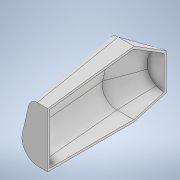
# Autodesk Inventor part: Housing
Saved by Autodesk Inventor 2021 (Build 250183000, 183)
## iProperties
Created: 2022-01-12
Part Number: Housing
Material: Generic
Document SubType Name: Modeling
Designer: stefi
Density: 1 g/cm^3
Appearance: Default
Author: stefi
Autodesk Inventor part; units mm, degrees
ref_plane "YZ Plane" through (0, 0, 0) normal (1, 0, 0) x (0, 1, 0)
ref_plane "XZ Plane" through (0, 0, 0) normal (0, 1, 0) x (-1, 0, 0)
ref_plane "Work Plane1" through (0, 0, 711.2) normal (0, 0, 1) x (1, 0, 0)
sketch "Sketch1" plane through (0, 0, 711.2) normal (0, 0, 1) x (1, 0, 0)
  line L0 (0.7413, 24.2751) -> (0.7413, -22.8249)
  line L1 (0.7413, -22.8249) -> (-11.3287, -22.8249)
  arc A0 (-23.0997, -8.085) -> (-11.3287, -22.8249) centre (-11.3287, -10.7549) ccw
  line L2 (-23.0997, -8.085) -> (-16.8814, 19.3297)
  arc A1 (-10.6887, 24.2751) -> (-16.8814, 19.3297) centre (-10.6887, 17.9251) ccw
  line L3 (-10.6887, 24.2751) -> (0.7413, 24.2751)
  point P0 (0, 0)
  dimension "d1" = 47.1
  dimension "d2" = 12.07
  dimension "d3" = 12.07
  dimension "d4" = 6.35
  dimension "d5" = 11.43
  constraints: 8 end point, 4 point on circle, 4 tangent, 2 centre point, 1 horizontal, 1 perpendicular, 1 vertical
  measures "d1" distance of L0.start L0.end
  measures "d2" distance of L0.end L1.end
  measures "d3" radius of A0
  measures "d4" radius of A1
  measures "d5" distance of L3.start L0.start
ref_plane "Work Plane2" through (0, 0, 773.2) normal (0, 0, 1) x (1, 0, 0)
sketch "Sketch2" plane through (0, 0, 773.2) normal (0, 0, 1) x (1, 0, 0)
  line L0 (0.7413, 16.5451) -> (0.7413, -22.8249)
  line L1 (0.7413, -22.8249) -> (-5.6087, -22.8249)
  arc A0 (-17.3671, -8.0297) -> (-5.6087, -22.8249) centre (-5.6087, -10.7549) ccw
  line L2 (-17.3671, -8.0297) -> (-12.8108, 11.6288)
  arc A1 (-6.6247, 16.5451) -> (-12.8108, 11.6288) centre (-6.6247, 10.1951) ccw
  line L3 (-6.6247, 16.5451) -> (0.7413, 16.5451)
  point P0 (0, 0)
  point P1 (0, 0)
  dimension "d7" = 39.37
  dimension "d8" = 6.35
  dimension "d9" = 12.07
  dimension "d10" = 6.35
  dimension "d11" = 7.366
  constraints: 8 end point, 4 point on circle, 4 tangent, 2 centre point, 1 horizontal, 1 perpendicular, 1 vertical
  measures "d7" distance of L0.start L0.end
  measures "d8" distance of L0.end L1.end
  measures "d9" radius of A0
  measures "d10" radius of A1
  measures "d11" distance of L3.start L0.start
loft "Loft1" add profiles "Sketch2", "Sketch1"
sketch "Sketch3" plane through (-6.6247, 16.5451, 773.2) normal (0, 0, 1) x (1, 0, 0)
  point P0 (6.6247, -16.5451)
ref_plane "Work Plane3" through (-6.6247, 16.5451, 688.2) normal (0, 0, 1) x (1, 0, 0)
sketch "Sketch4" plane through (-6.6247, 16.5451, 688.2) normal (0, 0, 1) x (1, 0, 0)
  line L0 (7.366, 0) -> (7.366, -39.37) projected
  arc A0 (7.366, -6.635) -> (7.366, -32.735) centre (7.366, -19.685) ccw
  point P0 (6.6247, -16.5451)
  dimension "d17" = 26.1
  constraints: 2 point on circle, 2 point on line, 1 centre point, 1 midpoint
  measures "d17" diameter of A0
loft "Loft2" add profiles "Sketch4" section 1 edges at (0.7413, 0.7251, 711.2) (-5.2937, -22.8249, 711.2) (-20.7604, -18.2868, 711.2) (-19.9906, 5.6223, 711.2) (-14.6512, 22.887, 711.2) (-4.9737, 24.2751, 711.2)
sketch "Sketch5" plane through (0.7413, -22.8249, 711.2) normal (1, 0, 0) x (0, 0, -1)
  point P0 (711.2, 22.8249)
sketch "Sketch6" plane through (0.7413, -22.8249, 773.2) normal (1, 0, 0) x (0, 0, -1)
  point P0 (773.2, 22.8249)
sketch "Sketch7" plane through (0.7413, -22.8249, 773.2) normal (1, 0, 0) x (0, 0, -1)
  point P0 (773.2, 22.8249)
shell "Shell1" thickness 1.54 removed faces 1 at (0.7413, 5.9984, 731.8667)
body "Solid1"
